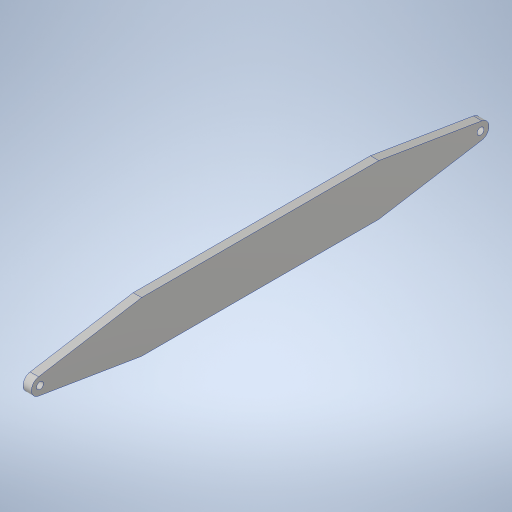
# Autodesk Inventor part: EL2-013
Saved by Autodesk Inventor 2023.4 (Build 274418000, 418)
## iProperties
Created: 2025-01-13
Part Number: EL2-013
Material: Aluminum 6061
Document SubType Name: Modeling
Designer: mavericks
Density: 2.7 g/cm^3
Appearance: Aluminum - Flat
Author: mavericks
Autodesk Inventor part; units mm, degrees
ref_plane "YZ Plane" through (0, 0, 0) normal (1, 0, 0) x (0, 1, 0)
ref_plane "XZ Plane" through (0, 0, 0) normal (0, 1, 0) x (-1, 0, 0)
ref_plane "XY Plane" through (0, 0, 0) normal (0, 0, 1) x (1, 0, 0)
sketch "Sketch1" plane through (0, 0, 0) normal (1, 0, 0) x (0, 1, 0)
  line L0 (-19.05, -177.8) -> (19.05, -177.8)
  line L1 (19.05, -177.8) -> (19.05, 177.8)
  line L2 (19.05, 177.8) -> (-19.05, 177.8)
  line L3 (-19.05, 177.8) -> (-19.05, -177.8)
  line L4 (-19.05, -177.8) -> (19.05, 177.8) construction
  line L5 (19.05, -177.8) -> (-19.05, 177.8) construction
  circle A0 centre (0, 165.1) radius 6.35 construction
  circle A1 centre (0, -165.1) radius 6.35 construction
  line L6 (0, 165.1) -> (0, -165.1) construction
  line L7 (6.2647, 166.137) -> (19.05, 88.9)
  line L8 (-6.2647, 166.137) -> (-19.05, 88.9)
  line L9 (6.2647, -166.137) -> (19.05, -88.9)
  line L10 (-6.2647, -166.137) -> (-19.05, -88.9)
  arc A2 (6.2647, 166.137) -> (-6.2647, 166.137) centre (0, 165.1) ccw
  arc A3 (-6.2647, -166.137) -> (6.2647, -166.137) centre (0, -165.1) ccw
  point P0 (0, 0)
  point P1 (0, 0)
  dimension "d1" = 38.1
  dimension "d2" = 355.6
  dimension "d15" = 12.7
  dimension "d16" = 12.7
  dimension "d17" = 330.2
  dimension "d18" = 88.9
  dimension "d19" = 88.9
  constraints: 22 end point, 8 point on circle, 4 centre point, 4 point on line, 4 tangent, 3 coincident, 3 midpoint, 2 horizontal alignment, 2 parallel, 2 vertical alignment, 1 horizontal, 1 perpendicular, 1 vertical
  measures "d1" distance of L1.end L2.end
  measures "d2" distance of L0.end L1.end
  measures "d15" diameter of A0
  measures "d16" diameter of A1
  measures "d17" distance of L6.start L6.end
  measures "d18" vertical distance of point (0, 0) L7.end
  measures "d19" vertical distance of point (0, 0) L9.end
extrude "Extrusion1" add sketch "Sketch1" along normal blind 6.35 contours L3 L8 A2 L7 L1 L9 A3 L10
sketch "Sketch2" plane through (6.35, 0, 0) normal (1, 0, 0) x (0, 0, -1)
  line L0 (-177.8, 25.4) -> (-177.8, -25.4) construction
  line L1 (177.8, -25.4) -> (177.8, 25.4) construction
  line L2 (-165.1, 0) -> (165.1, 0) construction
  point P0 (0, 0)
  point P1 (0, 0)
  dimension "d7" = 330.2
  constraints: 2 end point, 2 horizontal alignment, 1 coincident, 1 horizontal, 1 midpoint
  measures "d7" distance of L2.start L2.end
hole "Hole1" at (6.35, 0, 165.1) at (6.35, 0, -165.1) direction (-1, 0, 0) diameter 5.1054 end through all clearance for "Flat Head Machine Screw (82)" size "#10" standard "Ansi Unified Screw Threads"
equation "\"d19\" = d18"
body "Solid1"
